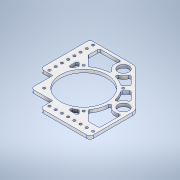
# Autodesk Inventor part: Plate_Bottom
Saved by Autodesk Inventor 2020 (Build 240168000, 168)
## iProperties
Created: 2019-05-28
Part Number: Plate_Bottom
Material: Aluminum 6061
Document SubType Name: Modeling
Designer: Connor
Density: 2.7 g/cm^3
Appearance: Aluminum - Flat
Author: Connor
Autodesk Inventor part; units mm, degrees
ref_plane "YZ Plane" through (0, 0, 0) normal (1, 0, 0) x (0, 1, 0)
ref_plane "XZ Plane" through (0, 0, 0) normal (0, 1, 0) x (-1, 0, 0)
ref_plane "XY Plane" through (0, 0, 0) normal (0, 0, 1) x (1, 0, 0)
sketch "Sketch1" plane through (0, 0, 0) normal (0, 1, 0) x (-1, 0, 0)
  line L0 (0, 0) -> (-190.5, 0)
  line L1 (-190.5, 0) -> (-190.5, -190.5)
  line L2 (-190.5, -190.5) -> (0, -190.5)
  line L3 (0, -190.5) -> (0, 0)
  circle A0 centre (-79.375, -79.375) radius 47.625
  line L4 (-25.4, -190.5) -> (-25.4, 0) construction
  line L5 (0, -25.4) -> (-190.5, -25.4) construction
  line L6 (0, 0) -> (-190.5, -190.5) construction
  circle A1 centre (-79.375, -79.375) radius 53.975 construction
  dimension "d0" = 95.25
  dimension "d3" = 25.4
  dimension "d4" = 25.4
  dimension "d5" = 107.95
  dimension "d48" = 165.1
  constraints: 14 end point, 7 point on line, 4 perpendicular, 2 centre point, 2 parallel, 1 coincident, 1 horizontal, 1 tangent
  measures "d0" diameter of A0
  measures "d3" distance between parallel lines of L0 L5
  measures "d4" distance between parallel lines of L3 L4
  measures "d5" diameter of A1
  measures "d48" distance between parallel lines of L5 L2
extrude "Extrusion1" add sketch "Sketch1" along normal blind 6.35
sketch "Sketch2" plane through (0, 6.35, 0) normal (0, 1, 0) x (1, 0, 0)
  circle A0 centre (79.375, 79.375) radius 47.625 construction
  circle A1 centre (79.375, 79.375) radius 57.15 construction
  line L0 (0, 190.5) -> (0, 0) construction
  arc A2 (177.8, 76.2) -> (76.2, 177.8) centre (76.2, 76.2) ccw construction
  line L1 (38.9638, 38.9638) -> (119.7862, 38.9638) construction
  line L2 (119.7862, 38.9638) -> (119.7862, 119.7862) construction
  line L3 (119.7862, 119.7862) -> (38.9638, 119.7862) construction
  line L4 (38.9638, 119.7862) -> (38.9638, 38.9638) construction
  dimension "d9" = 114.3
  constraints: 8 end point, 4 point on circle, 2 parallel, 2 perpendicular, 1 centre point, 1 coincident, 1 horizontal
  measures "d9" diameter of A1
hole "Hole1" at (38.9638, 6.35, -38.9638) at (119.7862, 6.35, -119.7862) at (119.7862, 6.35, -38.9638) at (38.9638, 6.35, -119.7862) direction (0, -1, 0) diameter 4.9784 end through all
sketch "Sketch4" plane through (0, 6.35, 0) normal (0, 1, 0) x (1, 0, 0)
  line L0 (0, 0) -> (190.5, 0) projected
  line L1 (0, 0) -> (25.4, 0)
  line L2 (25.4, 0) -> (25.4, 69.85)
  line L3 (25.4, 69.85) -> (0, 69.85)
  line L4 (0, 69.85) -> (0, 0)
  line L5 (25.4, 0) -> (69.85, 0)
  line L6 (69.85, 0) -> (69.85, 25.4)
  line L7 (69.85, 25.4) -> (25.4, 25.4)
  line L8 (25.4, 25.4) -> (25.4, 0)
  dimension "d26" = 25.4
  dimension "d27" = 69.85
  dimension "d28" = 44.45
  dimension "d29" = 25.4
  constraints: 16 end point, 4 parallel, 2 horizontal, 2 perpendicular
  measures "d26" distance of L3.end L2.end
  measures "d27" distance of L2.end L1.end
  measures "d28" distance of L7.end L6.end
  measures "d29" distance of L6.end L5.end
extrude "Extrusion3" cut sketch "Sketch4" against normal through all
sketch "Sketch5" plane through (0, 6.35, 0) normal (0, 1, 0) x (1, 0, 0)
  circle A0 centre (154.1438, 85.8655) radius 11.1125
  circle A1 centre (79.375, 79.375) radius 47.625 construction
  circle A2 centre (79.375, 79.375) radius 75.05 construction
  circle A3 centre (153.2048, 55.4) radius 25.4 construction
  circle A4 centre (119.7862, 38.9638) radius 2.4892 construction
  circle A5 centre (38.9638, 38.9638) radius 2.4892 construction
  circle A6 centre (119.7862, 119.7862) radius 2.4892 construction
  line L0 (38.9638, 38.9638) -> (119.7862, 119.7862) construction
  circle A7 centre (85.8655, 154.1438) radius 11.1125
  circle A8 centre (153.2048, 55.4) radius 7.62 construction
  circle A9 centre (154.1438, 85.8655) radius 22.86 construction
  line L1 (69.85, 0) -> (69.85, 25.4) construction
  line L2 (69.85, 25.4) -> (168.2375, 25.4) construction
  circle A10 centre (153.2048, 55.4) radius 30 construction
  circle A11 centre (153.2048, 55.4) radius 9.525
  circle A12 centre (55.4, 153.2048) radius 9.525
  circle A13 centre (79.375, 79.375) radius 47.625 projected
  point P0 (0, 0)
  dimension "d38" = 150.1
  dimension "d37" = 22.225
  dimension "d43" = 15.24
  dimension "d44" = 45.72
  dimension "d46" = 50.8
  dimension "d47" = 60
  dimension "d72" = 19.05
  constraints: 8 centre point, 5 coincident, 4 end point, 3 tangent, 2 symmetric about line, 1 horizontal, 5 other
  measures "d37" diameter of A0
  measures "d43" diameter of A8
  measures "d44" diameter of A9
  measures "d46" diameter of A3
  measures "d47" diameter of A10
  measures "d72" diameter of A11
extrude "Extrusion4" cut sketch "Sketch5" against normal through all contours A0 | A7
sketch "Sketch6" plane through (0, 6.35, 0) normal (0, 1, 0) x (1, 0, 0)
  line L0 (69.85, 0) -> (190.5, 0) projected
  line L1 (0, 190.5) -> (0, 69.85) projected
  point P0 (0, 0)
  point P1 (12.7, 12.7)
  point P2 (76.2, 0)
  point P3 (184.15, 0)
  point P4 (25.4, 12.7)
  point P5 (38.1, 12.7)
  point P6 (50.8, 12.7)
  point P7 (63.5, 12.7)
  point P8 (76.2, 12.7)
  point P9 (88.9, 12.7)
  point P10 (101.6, 12.7)
  point P11 (114.3, 12.7)
  point P12 (127, 12.7)
  point P13 (139.7, 12.7)
  point P14 (152.4, 12.7)
  point P15 (165.1, 12.7)
  point P16 (177.8, 12.7)
  point P17 (0, 184.15)
  point P18 (0, 76.2)
  point P19 (12.7, 25.4)
  point P20 (12.7, 38.1)
  point P21 (12.7, 50.8)
  point P22 (12.7, 63.5)
  point P23 (12.7, 76.2)
  point P24 (12.7, 88.9)
  point P25 (12.7, 101.6)
  point P26 (12.7, 114.3)
  point P27 (12.7, 127)
  point P28 (12.7, 139.7)
  point P29 (12.7, 152.4)
  point P30 (12.7, 165.1)
  point P31 (12.7, 177.8)
  dimension "d49" = 12.7
  dimension "d50" = 12.7
  dimension "d53" = 12.7
  dimension "d60" = 12.7
  constraints: 1 horizontal, 1 vertical, 26 other
  measures "d49" horizontal distance of point (0, 0) point (12.7, 12.7)
  measures "d50" horizontal distance of point (0, 0) point (12.7, 12.7)
  measures "d53" distance of point (12.7, 12.7) point (25.4, 12.7)
  measures "d60" distance of point (12.7, 12.7) point (12.7, 25.4)
hole "Hole2" at (12.7, 6.35, -12.7) at (25.4, 6.35, -12.7) at (38.1, 6.35, -12.7) at (50.8, 6.35, -12.7) at (63.5, 6.35, -12.7) at (76.2, 6.35, -12.7) at (88.9, 6.35, -12.7) at (101.6, 6.35, -12.7) at (114.3, 6.35, -12.7) at (127, 6.35, -12.7) at (139.7, 6.35, -12.7) at (152.4, 6.35, -12.7) at (165.1, 6.35, -12.7) at (177.8, 6.35, -12.7) at (12.7, 6.35, -25.4) at (12.7, 6.35, -38.1) at (12.7, 6.35, -50.8) at (12.7, 6.35, -63.5) at (12.7, 6.35, -76.2) at (12.7, 6.35, -88.9) at (12.7, 6.35, -101.6) at (12.7, 6.35, -114.3) at (12.7, 6.35, -127) at (12.7, 6.35, -139.7) at (12.7, 6.35, -152.4) at (12.7, 6.35, -165.1) at (12.7, 6.35, -177.8) direction (0, -1, 0) diameter 4.9784 end through all
sketch "Sketch8" plane through (0, 6.35, 0) normal (0, 1, 0) x (1, 0, 0)
  circle A0 centre (85.8655, 154.1438) radius 11.1125 projected
  circle A1 centre (85.8655, 154.1438) radius 17.4625
  circle A2 centre (154.1438, 85.8655) radius 11.1125 projected
  circle A3 centre (154.1438, 85.8655) radius 17.4625
  line L0 (85.8655, 171.6063) -> (0, 171.6063)
  line L1 (0, 190.5) -> (0, 69.85) projected
  line L2 (171.6063, 85.8655) -> (171.6063, 0)
  line L3 (69.85, 0) -> (190.5, 0) projected
  line L4 (98.2134, 166.4917) -> (166.4917, 98.2134)
  line L5 (190.5, 190.5) -> (0, 190.5) projected
  line L6 (190.5, 0) -> (190.5, 190.5) projected
  line L7 (28.575, 165.2563) -> (66.8155, 165.2563)
  arc A4 (69.7463, 160.8602) -> (76.9719, 139.1158) centre (85.8655, 154.1438) ccw
  circle A5 centre (79.375, 79.375) radius 47.625 projected
  circle A6 centre (38.9638, 119.7862) radius 2.4892 projected
  arc A7 (75.5782, 133.2163) -> (48.1037, 123.3683) centre (79.375, 79.375) ccw
  arc A8 (35.3817, 110.6463) -> (31.3972, 104.1022) centre (79.375, 79.375) ccw
  arc A9 (25.4, 105.5567) -> (31.3972, 104.1022) centre (28.575, 105.5567) ccw
  arc A10 (28.575, 165.2563) -> (25.4, 162.0813) centre (28.575, 162.0813) ccw
  arc A11 (69.7463, 160.8602) -> (66.8155, 165.2563) centre (66.8155, 162.0813) ccw
  arc A12 (75.5782, 133.2163) -> (76.9719, 139.1158) centre (75.3548, 136.3834) ccw
  arc A13 (44.0192, 123.7111) -> (48.1037, 123.3683) centre (46.2643, 125.9561) ccw
  arc A14 (35.3817, 110.6463) -> (35.0389, 114.7308) centre (32.7939, 112.4857) ccw
  line L8 (25.4, 69.85) -> (25.4, 25.4) projected
  line L9 (107.1936, 148.5312) -> (121.1272, 134.5976)
  line L10 (121.1272, 130.1075) -> (114.7308, 123.7111)
  arc A15 (110.6463, 123.3683) -> (92.3928, 131.7566) centre (79.375, 79.375) ccw
  arc A16 (92.0366, 137.8081) -> (102.0127, 147.495) centre (85.8655, 154.1438) ccw
  circle A17 centre (119.7862, 119.7862) radius 2.4892 construction
  line L11 (79.375, 79.375) -> (119.7862, 119.7862) construction
  arc A18 (92.0366, 137.8081) -> (92.3928, 131.7566) centre (93.1586, 134.8379) ccw
  arc A19 (107.1936, 148.5312) -> (102.0127, 147.495) centre (104.9486, 146.2861) ccw
  arc A20 (121.1272, 130.1075) -> (121.1272, 134.5976) centre (118.8821, 132.3525) ccw
  arc A21 (110.6463, 123.3683) -> (114.7308, 123.7111) centre (112.4857, 125.9561) ccw
  line L12 (148.5312, 107.1936) -> (134.5976, 121.1272)
  line L13 (130.1075, 121.1272) -> (123.7111, 114.7308)
  arc A22 (131.7566, 92.3928) -> (123.3683, 110.6463) centre (79.375, 79.375) ccw
  arc A23 (147.495, 102.0127) -> (137.8081, 92.0366) centre (154.1438, 85.8655) ccw
  arc A24 (131.7566, 92.3928) -> (137.8081, 92.0366) centre (134.8379, 93.1586) ccw
  arc A25 (147.495, 102.0127) -> (148.5312, 107.1936) centre (146.2861, 104.9486) ccw
  arc A26 (134.5976, 121.1272) -> (130.1075, 121.1272) centre (132.3525, 118.8821) ccw
  arc A27 (123.7111, 114.7308) -> (123.3683, 110.6463) centre (125.9561, 112.4857) ccw
  line L14 (35.0389, 114.7308) -> (30.8201, 118.9497)
  line L15 (44.0192, 123.7111) -> (26.3299, 141.4003)
  line L16 (79.375, 79.375) -> (38.9638, 119.7862) construction
  line L17 (25.4, 162.0813) -> (25.4, 143.6454)
  line L18 (25.4, 116.7046) -> (25.4, 105.5567)
  arc A28 (25.4, 143.6454) -> (26.3299, 141.4003) centre (28.575, 143.6454) ccw
  arc A29 (30.8201, 118.9497) -> (25.4, 116.7046) centre (28.575, 116.7046) ccw
  line L19 (165.2563, 28.575) -> (165.2563, 66.8155)
  arc A30 (139.1158, 76.9719) -> (160.8602, 69.7463) centre (154.1438, 85.8655) ccw
  arc A31 (123.3683, 48.1037) -> (133.2163, 75.5782) centre (79.375, 79.375) ccw
  arc A32 (104.1022, 31.3972) -> (110.6463, 35.3817) centre (79.375, 79.375) ccw
  arc A33 (104.1022, 31.3972) -> (105.5567, 25.4) centre (105.5567, 28.575) ccw
  arc A34 (162.0813, 25.4) -> (165.2563, 28.575) centre (162.0813, 28.575) ccw
  arc A35 (165.2563, 66.8155) -> (160.8602, 69.7463) centre (162.0813, 66.8155) ccw
  arc A36 (139.1158, 76.9719) -> (133.2163, 75.5782) centre (136.3834, 75.3548) ccw
  arc A37 (123.3683, 48.1037) -> (123.7111, 44.0192) centre (125.9561, 46.2643) ccw
  arc A38 (114.7308, 35.0389) -> (110.6463, 35.3817) centre (112.4857, 32.7939) ccw
  line L20 (114.7308, 35.0389) -> (118.9497, 30.8201)
  line L21 (123.7111, 44.0192) -> (141.4003, 26.3299)
  line L22 (162.0813, 25.4) -> (143.6454, 25.4)
  line L23 (116.7046, 25.4) -> (105.5567, 25.4)
  arc A39 (141.4003, 26.3299) -> (143.6454, 25.4) centre (143.6454, 28.575) ccw
  arc A40 (116.7046, 25.4) -> (118.9497, 30.8201) centre (116.7046, 28.575) ccw
  point P0 (0, 0)
  point P1 (160.8602, 69.7463)
  point P2 (139.1158, 76.9719)
  dimension "d94" = 34.925
  dimension "d98" = 3.175
  dimension "d99" = 6.35
  dimension "d102" = 6.35
  dimension "d103" = 6.35
  dimension "d105" = 6.35
  dimension "d108" = 6.35
  dimension "d109" = 6.35
  dimension "d113" = 6.35
  dimension "d114" = 6.35
  constraints: 72 point on circle, 38 end point, 38 symmetric about line, 36 centre point, 32 tangent, 12 equal radius, 7 coincident, 3 parallel, 2 collinear, 2 horizontal, 2 perpendicular, 2 point on line, 2 vertical, 17 other
  measures "d94" diameter of A1
  measures "d98" radius of A10
  measures "d99" distance between parallel lines of L0 L7
  measures "d102" radial gap between concentric circles of A5 A7
  measures "d103" radial gap between concentric circles of A5 A8
  measures "d105" distance between parallel lines of L4 L9
  measures "d108" radial gap between concentric circles of A5 A15
  measures "d109" distance between parallel lines of L11 L10
  measures "d113" distance between parallel lines of L16 L15
  measures "d114" distance between parallel lines of L16 L14
extrude "Extrusion6" cut sketch "Sketch8" against normal through all contours A1 L0 L1 L5 L6 L3 L2 A3 L4 | A19 L9 A20 L10 A21 A15 A18 A1 | A1 A12 A7 A13 L15 A28 L17 A10 L7 A11 | A3 A24 A22 A27 L13 A26 L12 A25 | A35 L19 A34 L22 A39 L21 A37 A31 A36 A3 | A8 A9 L18 A29 L14 A14 | A32 A38 L20 A40 L23 A33
fillet "Fillet7" radius 6.35 5 edges at (25.4, 3.175, -25.4) (69.85, 3.175, 0) (171.6063, 3.175, 0) (0, 3.175, -69.85) (0, 3.175, -171.6063)
body "Solid1"
